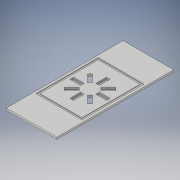
# Autodesk Inventor part: cuerpo-base-bateria
Saved by Autodesk Inventor 2019 (Build 230136000, 136)
## iProperties
Created: 2020-03-02
Part Number: cuerpo-base-bateria
Material: Generic
Document SubType Name: Modeling
Designer: jacqu
Density: 1 g/cm^3
Appearance: Default
Author: jacqu
Autodesk Inventor part; units mm, degrees
ref_plane "YZ Plane" through (0, 0, 0) normal (1, 0, 0) x (0, 1, 0)
ref_plane "XZ Plane" through (0, 0, 0) normal (0, 1, 0) x (-1, 0, 0)
ref_plane "XY Plane" through (0, 0, 0) normal (0, 0, 1) x (1, 0, 0)
sketch "Sketch7" plane through (0, 0, 0) normal (0, 1, 0) x (-1, 0, 0)
  circle A0 centre (-43.3, 100) radius 13.3 construction
  circle A1 centre (-43.3, 100) radius 31.3 construction
  line L0 (-86.6, 0) -> (0, 0)
  line L1 (0, 0) -> (0, 200)
  line L2 (0, 200) -> (-86.6, 200)
  line L3 (-86.6, 200) -> (-86.6, 0)
  line L4 (0, 200) -> (-86.6, 200)
  line L5 (-46.3, 68.8441) -> (-46.3, 87.0428)
  line L6 (-40.3, 68.8441) -> (-40.3, 87.0428)
  arc A2 (-46.3, 87.0428) -> (-40.3, 87.0428) centre (-43.3, 100) ccw
  arc A3 (-46.3, 68.8441) -> (-40.3, 68.8441) centre (-43.3, 100) ccw
  line L7 (-19.1481, 80.0908) -> (-32.0165, 92.9592)
  arc A4 (-23.3908, 75.8481) -> (-19.1481, 80.0908) centre (-43.3, 100) ccw
  line L8 (-23.3908, 75.8481) -> (-36.2592, 88.7165)
  arc A5 (-36.2592, 88.7165) -> (-32.0165, 92.9592) centre (-43.3, 100) ccw
  line L9 (-12.1441, 103) -> (-30.3428, 103)
  arc A6 (-12.1441, 97) -> (-12.1441, 103) centre (-43.3, 100) ccw
  line L10 (-12.1441, 97) -> (-30.3428, 97)
  arc A7 (-30.3428, 97) -> (-30.3428, 103) centre (-43.3, 100) ccw
  line L11 (-23.3908, 124.1519) -> (-36.2592, 111.2835)
  arc A8 (-19.1481, 119.9092) -> (-23.3908, 124.1519) centre (-43.3, 100) ccw
  line L12 (-19.1481, 119.9092) -> (-32.0165, 107.0408)
  arc A9 (-32.0165, 107.0408) -> (-36.2592, 111.2835) centre (-43.3, 100) ccw
  line L13 (-46.3, 131.1559) -> (-46.3, 112.9572)
  arc A10 (-40.3, 131.1559) -> (-46.3, 131.1559) centre (-43.3, 100) ccw
  line L14 (-40.3, 131.1559) -> (-40.3, 112.9572)
  arc A11 (-40.3, 112.9572) -> (-46.3, 112.9572) centre (-43.3, 100) ccw
  line L15 (-67.4519, 119.9092) -> (-54.5835, 107.0408)
  arc A12 (-63.2092, 124.1519) -> (-67.4519, 119.9092) centre (-43.3, 100) ccw
  line L16 (-63.2092, 124.1519) -> (-50.3408, 111.2835)
  arc A13 (-50.3408, 111.2835) -> (-54.5835, 107.0408) centre (-43.3, 100) ccw
  line L17 (-74.4559, 97) -> (-56.2572, 97)
  arc A14 (-74.4559, 103) -> (-74.4559, 97) centre (-43.3, 100) ccw
  line L18 (-74.4559, 103) -> (-56.2572, 103)
  arc A15 (-56.2572, 103) -> (-56.2572, 97) centre (-43.3, 100) ccw
  line L19 (-63.2092, 75.8481) -> (-50.3408, 88.7165)
  arc A16 (-67.4519, 80.0908) -> (-63.2092, 75.8481) centre (-43.3, 100) ccw
  line L20 (-67.4519, 80.0908) -> (-54.5835, 92.9592)
  arc A17 (-54.5835, 92.9592) -> (-50.3408, 88.7165) centre (-43.3, 100) ccw
  line L21 (-86.6, 200) -> (-86.6, 0)
  point P0 (-43.3, 200)
  point P1 (-86.6, 100)
  point P2 (-43.3, 200)
  point P3 (-43.3, 86.7)
  point P4 (-33.8955, 90.5955)
  point P5 (-30, 100)
  point P6 (-33.8955, 109.4045)
  point P7 (-43.3, 113.3)
  point P8 (-52.7045, 109.4045)
  point P9 (-56.6, 100)
  point P10 (-52.7045, 90.5955)
  dimension "d36" = 18
  dimension "d37" = 6
  dimension "d38" = 360
  dimension "d39" = 30
  dimension "d42" = 100
  dimension "d43" = 200
  dimension "d44" = 86.6
  constraints: 44 end point, 37 point on circle, 18 centre point, 4 parallel, 3 midpoint, 3 vertical alignment, 2 coincident, 2 concentric, 1 horizontal alignment, 1 vertical, 89 other
  measures "d36" radial gap between concentric circles of A1 A0
  measures "d37" distance between parallel lines of L6 L5
  measures "d39" distance of point (-86.6, 100) point (-56.6, 100)
  measures "d42" distance from line of L2 A0.centre
  measures "d43" distance of L0.end L1.end
  measures "d44" distance of L1.end L2.end
extrude "Extrusion3" add sketch "Sketch7" along normal blind 3.3
sketch "Sketch8" plane through (0, 3.3, 0) normal (0, 1, 0) x (1, 0, 0)
  line L0 (7.3, -150.05) -> (79.3, -150.05)
  line L1 (79.3, -150.05) -> (79.3, -49.95)
  line L2 (79.3, -49.95) -> (7.3, -49.95)
  line L3 (7.3, -49.95) -> (7.3, -150.05)
  line L4 (4.1, -153.25) -> (82.5, -153.25)
  line L5 (82.5, -153.25) -> (82.5, -46.75)
  line L6 (82.5, -46.75) -> (4.1, -46.75)
  line L7 (4.1, -46.75) -> (4.1, -153.25)
  line L8 (86.6, 0) -> (0, 0) projected
  line L9 (0, 0) -> (0, -200) projected
  dimension "d47" = 3.2
  dimension "d48" = 3.2
  dimension "d49" = 3.2
  dimension "d50" = 3.2
  dimension "largo_bateria" = 100.1
  dimension "ancho_bateria" = 72
  dimension "d54" = 7.3
  dimension "d55" = 49.95
  constraints: 16 end point, 4 parallel, 2 horizontal, 2 perpendicular
  measures "d47" distance between parallel lines of L0 L4
  measures "d48" distance between parallel lines of L7 L3
  measures "d49" distance between parallel lines of L6 L2
  measures "d50" distance between parallel lines of L5 L1
  measures "largo_bateria" distance of L2.end L0.start
  measures "ancho_bateria" distance of L0.start L0.end
  measures "d54" distance between parallel lines of L3 L9
  measures "d55" distance between parallel lines of L2 L8
extrude "Extrusion4" cut sketch "Sketch8" against normal blind 1
equation "\"d36\" = 1.5 * d41"
equation "\"d37\" = 0.2 * d39"
equation "\"d39\" = d40"
equation "\"d42\" = 0.5 * largo_base"
equation "\"d43\" = largo_base"
equation "\"d48\" = d47"
equation "\"d49\" = d47"
equation "\"d50\" = d47"
equation "\"d55\" = 0.5 * largo_base - 0.5 * largo_bateria"
equation "\"espesor\" = 3.2"
equation "\"d41\" = 12"
equation "\"largo_base\" = 200"
equation "\"d40\" = 30"
body "Solid2"
